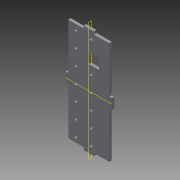
# Autodesk Inventor part: baseBoxLongSide01
Saved by Autodesk Inventor 2013 (Build 170138000, 138)
## iProperties
Created: 2014-10-07
Part Number: baseBoxLongSide01
Material: Generic
Document SubType Name: Modeling
Designer: Nano
Density: 1 g/cm^3
Author: Nano
Autodesk Inventor part; units mm, degrees
ref_plane "YZ Plane" through (0, 0, 0) normal (1, 0, 0) x (0, 1, 0)
ref_plane "XZ Plane" through (0, 0, 0) normal (0, 1, 0) x (-1, 0, 0)
ref_plane "XY Plane" through (0, 0, 0) normal (0, 0, 1) x (1, 0, 0)
sketch "Sketch1" plane through (0, 0, 0) normal (0, 0, 1) x (1, 0, 0)
  line L0 (-101.6, -273.05) -> (-101.6, 6.35) projected
  line L1 (0, -273.05) -> (0, 6.35) projected
  line L2 (0, -6.35) -> (-101.6, -6.35) projected
  line L3 (0, -260.35) -> (-101.6, -260.35) projected
  point P0 (0, 0)
extrude "Extrusion1" add sketch "Sketch1" against normal blind 6.35
sketch "Sketch2" plane through (-101.6, -260.35, 0) normal (0, -1, 0) x (1, 0, 0)
  line L0 (0, 0) -> (0, -6.35) projected
  line L1 (101.6, 0) -> (101.6, -6.35) projected
  line L2 (38.1, 0) -> (63.5, 0)
  line L3 (63.5, 0) -> (63.5, -6.35)
  line L4 (63.5, -6.35) -> (38.1, -6.35)
  line L5 (38.1, -6.35) -> (38.1, 0)
  dimension "d2" = 25.4
  dimension "d3" = 38.1
  dimension "d4" = 38.1
  constraints: 8 end point, 2 parallel, 1 horizontal, 1 perpendicular
  measures "d2" distance of L3.end L4.end
  measures "d3" distance between parallel lines of L0 L5
  measures "d4" distance between parallel lines of L1 L3
extrude "Extrusion2" add sketch "Sketch2" along normal blind 6.35
ref_plane "Work Plane1" through (-101.6, -133.35, -6.35) normal (0, -1, 0) x (1, 0, 0)
mirror "Mirror1" about plane through (-101.6, -133.35, -6.35) normal (0, -1, 0) of "Extrusion2"
sketch "Sketch3" plane through (0, -260.35, 0) normal (1, 0, 0) x (0, 0, -1)
  line L0 (0, 0) -> (6.35, 0) projected
  line L1 (0, 254) -> (6.35, 254) projected
  line L2 (0, 139.7) -> (6.35, 139.7)
  line L3 (6.35, 139.7) -> (6.35, 114.3)
  line L4 (6.35, 114.3) -> (0, 114.3)
  line L5 (0, 114.3) -> (0, 139.7)
  point P0 (0, 260.35)
  dimension "d7" = 25.4
  dimension "d8" = 6.35
  dimension "d9" = 114.3
  dimension "d10" = 114.3
  constraints: 8 end point, 2 parallel, 1 horizontal, 1 perpendicular
  measures "d7" distance of L2.end L3.end
  measures "d8" distance of L2.start L2.end
  measures "d9" distance between parallel lines of L1 L2
  measures "d10" distance between parallel lines of L0 L4
extrude "Extrusion3" add sketch "Sketch3" along normal blind 6.35
ref_plane "Work Plane2" through (-50.8, -260.35, 0) normal (1, 0, 0) x (0, 0, -1)
mirror "Mirror2" about plane through (-50.8, -260.35, 0) normal (1, 0, 0) of "Extrusion3"
sketch "Sketch4" plane through (0, 0, 0) normal (0, 0, 1) x (1, 0, 0)
  line L0 (0, -6.35) -> (0, -120.65) projected
  line L1 (-38.1, -6.35) -> (0, -6.35) projected
  line L2 (-25.4, -50.8) -> (-50.8, -50.8)
  line L3 (-50.8, -50.8) -> (-50.8, -76.2)
  line L4 (-50.8, -76.2) -> (-25.4, -76.2)
  line L5 (-25.4, -76.2) -> (-25.4, -50.8)
  point P0 (0, 0)
  dimension "d13" = 25.4
  dimension "d14" = 25.4
  dimension "d15" = 25.4
  dimension "d16" = 44.45
  constraints: 8 end point, 2 parallel, 1 horizontal, 1 perpendicular
  measures "d13" distance of L4.end L3.end
  measures "d14" distance of L3.end L2.end
  measures "d15" distance between parallel lines of L5 L0
  measures "d16" distance between parallel lines of L1 L2
extrude "Extrusion4" cut sketch "Sketch4" against normal through all
sketch "Sketch5" plane through (0, 0, 0) normal (0, 0, 1) x (1, 0, 0)
  line L0 (-101.6, -6.35) -> (-63.5, -6.35) projected
  line L1 (-101.6, -120.65) -> (-101.6, -6.35) projected
  line L2 (0, -260.35) -> (-38.1, -260.35) projected
  circle A0 centre (-83.82, -19.05) radius 3.9687
  circle A1 centre (-83.82, -57.15) radius 3.9687
  circle A2 centre (-83.82, -95.25) radius 3.9687
  circle A3 centre (-83.82, -133.35) radius 3.9687
  circle A4 centre (-83.82, -171.45) radius 3.9687
  circle A5 centre (-83.82, -209.55) radius 3.9687
  circle A6 centre (-83.82, -247.65) radius 3.9687
  circle A7 centre (-45.72, -19.05) radius 3.9687
  circle A8 centre (-45.72, -95.25) radius 3.9687
  circle A9 centre (-45.72, -133.35) radius 3.9687
  circle A10 centre (-45.72, -171.45) radius 3.9687
  circle A11 centre (-45.72, -209.55) radius 3.9687
  circle A12 centre (-45.72, -247.65) radius 3.9687
  point P0 (0, 0)
  dimension "d19" = 7.9375
  dimension "d20" = 17.78
  dimension "d21" = 12.7
  dimension "d24" = 38.1
  dimension "d31" = 38.1
  constraints: 13 centre point, 1 horizontal, 1 vertical, 24 other
  measures "d19" diameter of A0
  measures "d20" distance from line of A0.centre L1
  measures "d21" distance from line of L0 A0.centre
  measures "d24" distance of A0.centre A1.centre
  measures "d31" distance of A2.centre A8.centre
extrude "Extrusion5" cut sketch "Sketch5" against normal through all
equation "\"d3\" = d4"
equation "\"d9\" = d10"
body "Solid1"
